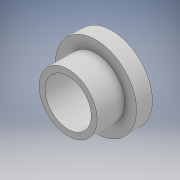
# Autodesk Inventor part: CapForCl
Saved by Autodesk Inventor 2017.3 (Build 213256000, 256)
## iProperties
Created: 2017-07-24
Part Number: CapForCl
Material: Generic
Document SubType Name: Modeling
Designer: steele
Density: 1 g/cm^3
Appearance: Default
Author: steele
Autodesk Inventor part; units mm, degrees
ref_plane "YZ Plane" through (0, 0, 0) normal (1, 0, 0) x (0, 1, 0)
ref_plane "XZ Plane" through (0, 0, 0) normal (0, 1, 0) x (-1, 0, 0)
ref_plane "XY Plane" through (0, 0, 0) normal (0, 0, 1) x (1, 0, 0)
sketch "Sketch2" plane through (0, 0, 0) normal (0, 0, 1) x (1, 0, 0)
  line L0 (0, 0) -> (0, 9.05) construction
  line L1 (0, 9.05) -> (-8.4, 9.05)
  line L2 (-8.4, 9.05) -> (-8.4, 5.75)
  line L3 (-8.4, 5.75) -> (-6, 5.75)
  line L4 (-6, 5.75) -> (-6, 0)
  line L5 (-6, 0) -> (-4.7743, 0)
  line L6 (0, 0) -> (-6, 0) construction
  line L7 (-4.7743, 0) -> (-4.7743, 6)
  line L8 (0, 9.05) -> (0, 8.5)
  line L9 (-4.7743, 8.5) -> (-4.7743, 6)
  line L10 (-4.7743, 8.5) -> (0, 8.5)
  dimension "d4" = 8.4
  dimension "d5" = 3.3
  dimension "d6" = 5.75
  dimension "d8" = 6
  constraints: 22 end point, 5 perpendicular, 3 vertical, 2 point on line, 1 collinear, 1 horizontal, 1 parallel
  measures "d4" distance of L0.end L1.end
  measures "d5" distance of L1.end L2.end
  measures "d6" distance of L3.end L4.end
  measures "d8" distance between parallel lines of L0 L4
revolve "Revolution1" add sketch "Sketch2" angle 360 about axis through (0, 0, 0) along (0, 1, 0)
body "Solid1"
